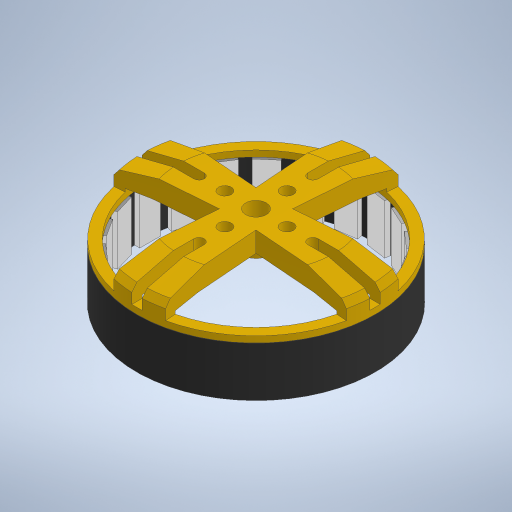
# Autodesk Inventor part: CAN
Saved by Autodesk Inventor 2023.1 (Build 271208000, 208)
## iProperties
Created: 2022-11-08
Part Number: CAN
Material: Generic
Document SubType Name: Modeling
Designer: Nathan Cai
Density: 1 g/cm^3
Appearance: Default
Author: Nathan Cai
Autodesk Inventor part; units mm, degrees
ref_plane "YZ Plane" through (0, 0, 0) normal (1, 0, 0) x (0, 1, 0)
ref_plane "XZ Plane" through (0, 0, 0) normal (0, 1, 0) x (-1, 0, 0)
ref_plane "XY Plane" through (0, 0, 0) normal (0, 0, 1) x (1, 0, 0)
sketch "Sketch1" plane through (0, 0, 0) normal (0, 1, 0) x (-1, 0, 0)
  circle A0 centre (0, 0) radius 23.05
  circle A1 centre (0, 0) radius 21.55
  line L0 (23.05, 0) -> (0, 0) construction
  dimension "d0" = 46.1
  dimension "d1" = 1.5
  constraints: 2 coincident, 2 end point, 1 centre point, 1 horizontal, 1 horizontal alignment, 2 other
extrude "Extrusion1" add sketch "Sketch1" along normal blind 9.6
sketch "Sketch2" plane through (0, 0, 0) normal (0, -1, 0) x (1, 0, 0)
  circle A0 centre (0, 0) radius 21.55 construction
  line L0 (21.55, 0) -> (0, 0) construction
  line L1 (20.457, 2) -> (21.457, 2)
  line L2 (21.457, 2) -> (21.457, -2)
  line L3 (21.457, -2) -> (20.457, -2)
  line L4 (20.457, -2) -> (20.457, 2)
  line L5 (20.457, 2) -> (21.457, -2) construction
  line L6 (21.457, 2) -> (20.457, -2) construction
  line L7 (19.0649, 7.6824) -> (20.0244, 7.9641)
  line L8 (20.0244, 7.9641) -> (21.1513, 4.1261)
  line L9 (21.1513, 4.1261) -> (20.1918, 3.8444)
  line L10 (20.1918, 3.8444) -> (19.0649, 7.6824)
  line L11 (19.0649, 7.6824) -> (21.1513, 4.1261) construction
  line L12 (20.0244, 7.9641) -> (20.1918, 3.8444) construction
  line L13 (16.1282, 12.7424) -> (16.9695, 13.283)
  line L14 (16.9695, 13.283) -> (19.1321, 9.918)
  line L15 (19.1321, 9.918) -> (18.2908, 9.3774)
  line L16 (18.2908, 9.3774) -> (16.1282, 12.7424)
  line L17 (16.1282, 12.7424) -> (19.1321, 9.918) construction
  line L18 (16.9695, 13.283) -> (18.2908, 9.3774) construction
  line L19 (11.885, 16.7701) -> (12.5398, 17.5258)
  line L20 (12.5398, 17.5258) -> (15.5628, 14.9064)
  line L21 (15.5628, 14.9064) -> (14.908, 14.1506)
  line L22 (14.908, 14.1506) -> (11.885, 16.7701)
  line L23 (11.885, 16.7701) -> (15.5628, 14.9064) construction
  line L24 (12.5398, 17.5258) -> (14.908, 14.1506) construction
  line L25 (6.6789, 19.4392) -> (7.0943, 20.3488)
  line L26 (7.0943, 20.3488) -> (10.7328, 18.6871)
  line L27 (10.7328, 18.6871) -> (10.3174, 17.7775)
  line L28 (10.3174, 17.7775) -> (6.6789, 19.4392)
  line L29 (6.6789, 19.4392) -> (10.7328, 18.6871) construction
  line L30 (7.0943, 20.3488) -> (10.3174, 17.7775) construction
  line L31 (0.9317, 20.5334) -> (1.074, 21.5232)
  line L32 (1.074, 21.5232) -> (5.0333, 20.954)
  line L33 (5.0333, 20.954) -> (4.891, 19.9641)
  line L34 (4.891, 19.9641) -> (0.9317, 20.5334)
  line L35 (0.9317, 20.5334) -> (5.0333, 20.954) construction
  line L36 (1.074, 21.5232) -> (4.891, 19.9641) construction
  line L37 (-4.891, 19.9641) -> (-5.0333, 20.954)
  line L38 (-5.0333, 20.954) -> (-1.074, 21.5232)
  line L39 (-1.074, 21.5232) -> (-0.9317, 20.5334)
  line L40 (-0.9317, 20.5334) -> (-4.891, 19.9641)
  line L41 (-4.891, 19.9641) -> (-1.074, 21.5232) construction
  line L42 (-5.0333, 20.954) -> (-0.9317, 20.5334) construction
  line L43 (-10.3174, 17.7775) -> (-10.7328, 18.6871)
  line L44 (-10.7328, 18.6871) -> (-7.0943, 20.3488)
  line L45 (-7.0943, 20.3488) -> (-6.6789, 19.4392)
  line L46 (-6.6789, 19.4392) -> (-10.3174, 17.7775)
  line L47 (-10.3174, 17.7775) -> (-7.0943, 20.3488) construction
  line L48 (-10.7328, 18.6871) -> (-6.6789, 19.4392) construction
  line L49 (-14.908, 14.1506) -> (-15.5628, 14.9064)
  line L50 (-15.5628, 14.9064) -> (-12.5398, 17.5258)
  line L51 (-12.5398, 17.5258) -> (-11.885, 16.7701)
  line L52 (-11.885, 16.7701) -> (-14.908, 14.1506)
  line L53 (-14.908, 14.1506) -> (-12.5398, 17.5258) construction
  line L54 (-15.5628, 14.9064) -> (-11.885, 16.7701) construction
  line L55 (-18.2908, 9.3774) -> (-19.1321, 9.918)
  line L56 (-19.1321, 9.918) -> (-16.9695, 13.283)
  line L57 (-16.9695, 13.283) -> (-16.1282, 12.7424)
  line L58 (-16.1282, 12.7424) -> (-18.2908, 9.3774)
  line L59 (-18.2908, 9.3774) -> (-16.9695, 13.283) construction
  line L60 (-19.1321, 9.918) -> (-16.1282, 12.7424) construction
  line L61 (-20.1918, 3.8444) -> (-21.1513, 4.1261)
  line L62 (-21.1513, 4.1261) -> (-20.0244, 7.9641)
  line L63 (-20.0244, 7.9641) -> (-19.0649, 7.6824)
  line L64 (-19.0649, 7.6824) -> (-20.1918, 3.8444)
  line L65 (-20.1918, 3.8444) -> (-20.0244, 7.9641) construction
  line L66 (-21.1513, 4.1261) -> (-19.0649, 7.6824) construction
  line L67 (-20.457, -2) -> (-21.457, -2)
  line L68 (-21.457, -2) -> (-21.457, 2)
  line L69 (-21.457, 2) -> (-20.457, 2)
  line L70 (-20.457, 2) -> (-20.457, -2)
  line L71 (-20.457, -2) -> (-21.457, 2) construction
  line L72 (-21.457, -2) -> (-20.457, 2) construction
  line L73 (-19.0649, -7.6824) -> (-20.0244, -7.9641)
  line L74 (-20.0244, -7.9641) -> (-21.1513, -4.1261)
  line L75 (-21.1513, -4.1261) -> (-20.1918, -3.8444)
  line L76 (-20.1918, -3.8444) -> (-19.0649, -7.6824)
  line L77 (-19.0649, -7.6824) -> (-21.1513, -4.1261) construction
  line L78 (-20.0244, -7.9641) -> (-20.1918, -3.8444) construction
  line L79 (-16.1282, -12.7424) -> (-16.9695, -13.283)
  line L80 (-16.9695, -13.283) -> (-19.1321, -9.918)
  line L81 (-19.1321, -9.918) -> (-18.2908, -9.3774)
  line L82 (-18.2908, -9.3774) -> (-16.1282, -12.7424)
  line L83 (-16.1282, -12.7424) -> (-19.1321, -9.918) construction
  line L84 (-16.9695, -13.283) -> (-18.2908, -9.3774) construction
  line L85 (-11.885, -16.7701) -> (-12.5398, -17.5258)
  line L86 (-12.5398, -17.5258) -> (-15.5628, -14.9064)
  line L87 (-15.5628, -14.9064) -> (-14.908, -14.1506)
  line L88 (-14.908, -14.1506) -> (-11.885, -16.7701)
  line L89 (-11.885, -16.7701) -> (-15.5628, -14.9064) construction
  line L90 (-12.5398, -17.5258) -> (-14.908, -14.1506) construction
  line L91 (-6.6789, -19.4392) -> (-7.0943, -20.3488)
  line L92 (-7.0943, -20.3488) -> (-10.7328, -18.6871)
  line L93 (-10.7328, -18.6871) -> (-10.3174, -17.7775)
  line L94 (-10.3174, -17.7775) -> (-6.6789, -19.4392)
  line L95 (-6.6789, -19.4392) -> (-10.7328, -18.6871) construction
  line L96 (-7.0943, -20.3488) -> (-10.3174, -17.7775) construction
  line L97 (-0.9317, -20.5334) -> (-1.074, -21.5232)
  line L98 (-1.074, -21.5232) -> (-5.0333, -20.954)
  line L99 (-5.0333, -20.954) -> (-4.891, -19.9641)
  line L100 (-4.891, -19.9641) -> (-0.9317, -20.5334)
  line L101 (-0.9317, -20.5334) -> (-5.0333, -20.954) construction
  line L102 (-1.074, -21.5232) -> (-4.891, -19.9641) construction
  line L103 (4.891, -19.9641) -> (5.0333, -20.954)
  line L104 (5.0333, -20.954) -> (1.074, -21.5232)
  line L105 (1.074, -21.5232) -> (0.9317, -20.5334)
  line L106 (0.9317, -20.5334) -> (4.891, -19.9641)
  line L107 (4.891, -19.9641) -> (1.074, -21.5232) construction
  line L108 (5.0333, -20.954) -> (0.9317, -20.5334) construction
  line L109 (10.3174, -17.7775) -> (10.7328, -18.6871)
  line L110 (10.7328, -18.6871) -> (7.0943, -20.3488)
  line L111 (7.0943, -20.3488) -> (6.6789, -19.4392)
  line L112 (6.6789, -19.4392) -> (10.3174, -17.7775)
  line L113 (10.3174, -17.7775) -> (7.0943, -20.3488) construction
  line L114 (10.7328, -18.6871) -> (6.6789, -19.4392) construction
  line L115 (14.908, -14.1506) -> (15.5628, -14.9064)
  line L116 (15.5628, -14.9064) -> (12.5398, -17.5258)
  line L117 (12.5398, -17.5258) -> (11.885, -16.7701)
  line L118 (11.885, -16.7701) -> (14.908, -14.1506)
  line L119 (14.908, -14.1506) -> (12.5398, -17.5258) construction
  line L120 (15.5628, -14.9064) -> (11.885, -16.7701) construction
  line L121 (18.2908, -9.3774) -> (19.1321, -9.918)
  line L122 (19.1321, -9.918) -> (16.9695, -13.283)
  line L123 (16.9695, -13.283) -> (16.1282, -12.7424)
  line L124 (16.1282, -12.7424) -> (18.2908, -9.3774)
  line L125 (18.2908, -9.3774) -> (16.9695, -13.283) construction
  line L126 (19.1321, -9.918) -> (16.1282, -12.7424) construction
  line L127 (20.1918, -3.8444) -> (21.1513, -4.1261)
  line L128 (21.1513, -4.1261) -> (20.0244, -7.9641)
  line L129 (20.0244, -7.9641) -> (19.0649, -7.6824)
  line L130 (19.0649, -7.6824) -> (20.1918, -3.8444)
  line L131 (20.1918, -3.8444) -> (20.0244, -7.9641) construction
  line L132 (21.1513, -4.1261) -> (19.0649, -7.6824) construction
  point P0 (20.957, 0)
  point P1 (20.6771, 6.0713)
  point P2 (20.1081, 5.9043)
  point P3 (18.129, 11.6508)
  point P4 (17.6301, 11.3302)
  point P5 (14.1122, 16.2864)
  point P6 (13.7239, 15.8382)
  point P7 (8.9522, 19.6026)
  point P8 (8.7058, 19.0632)
  point P9 (3.0669, 21.3307)
  point P10 (2.9825, 20.7437)
  point P11 (-3.0669, 21.3307)
  point P12 (-2.9825, 20.7437)
  point P13 (-8.9522, 19.6026)
  point P14 (-8.7058, 19.0632)
  point P15 (-14.1122, 16.2864)
  point P16 (-13.7239, 15.8382)
  point P17 (-18.129, 11.6508)
  point P18 (-17.6301, 11.3302)
  point P19 (-20.6771, 6.0713)
  point P20 (-20.1081, 5.9043)
  point P21 (-21.55, 0)
  point P22 (-20.957, 0)
  point P23 (-20.6771, -6.0713)
  point P24 (-20.1081, -5.9043)
  point P25 (-18.129, -11.6508)
  point P26 (-17.6301, -11.3302)
  point P27 (-14.1122, -16.2864)
  point P28 (-13.7239, -15.8382)
  point P29 (-8.9522, -19.6026)
  point P30 (-8.7058, -19.0632)
  point P31 (-3.0669, -21.3307)
  point P32 (-2.9825, -20.7437)
  point P33 (3.0669, -21.3307)
  point P34 (2.9825, -20.7437)
  point P35 (8.9522, -19.6026)
  point P36 (8.7058, -19.0632)
  point P37 (14.1122, -16.2864)
  point P38 (13.7239, -15.8382)
  point P39 (18.129, -11.6508)
  point P40 (17.6301, -11.3302)
  point P41 (20.6771, -6.0713)
  point P42 (20.1081, -5.9043)
  dimension "d4" = 1
  dimension "d5" = 4
  dimension "d8" = 360
  constraints: 266 end point, 2 horizontal, 2 midpoint, 2 parallel, 2 point on circle, 1 perpendicular, 1 point on line, 265 other
  measures "d4" distance of L2.end L3.end
  measures "d5" distance of L1.end L2.end
extrude "Extrusion2" add sketch "Sketch2" against normal blind 9.6
sketch "Sketch4" plane through (0, 0, 0) normal (1, 0, 0) x (0, 1, 0)
  line L0 (9.6, 2) -> (9.6, -2) projected
  line L1 (9.6, 0) -> (15.8, 0)
  line L2 (15.8, 0) -> (15.8, 23)
  line L3 (15.8, 23) -> (9.6, 23)
  line L4 (9.6, 23) -> (9.6, 0)
  line L5 (9.6, 0) -> (11.9, 0)
  line L6 (11.9, 0) -> (11.9, 21)
  line L7 (11.9, 21) -> (9.6, 21)
  line L8 (9.6, 21) -> (9.6, 0)
  line L9 (11.4, 21) -> (11.9, 16.3)
  line L10 (9.6, 0) -> (15.8, 0)
  line L11 (15.8, 0) -> (15.8, 3)
  line L12 (15.8, 3) -> (9.6, 3) construction
  line L13 (9.6, 3) -> (9.6, 0)
  line L14 (9.6, 3) -> (11.9, 3.75)
  line L15 (15.8, 0) -> (9.6, 0)
  line L16 (9.6, 0) -> (9.6, 2)
  line L17 (9.6, 2) -> (15.8, 2)
  line L18 (15.8, 2) -> (15.8, 0)
  point P0 (0, 0)
  dimension "d15" = 6.2
  dimension "d16" = 23
  dimension "d17" = 2.3
  dimension "d18" = 21
  dimension "d19" = 1.8
  dimension "d20" = 4.7
  dimension "d28" = 3
  dimension "d29" = 3.75
  dimension "d30" = 2
  constraints: 36 end point, 8 parallel, 4 horizontal, 4 perpendicular, 4 point on line, 1 midpoint
  measures "d15" distance of L3.end L2.end
  measures "d16" distance of L2.end L1.end
  measures "d17" distance of L7.end L6.end
  measures "d18" distance of L6.end L5.end
  measures "d19" distance from line of L4 L9.start
  measures "d20" distance from line of L7 L9.end
  measures "d28" distance of L11.end L10.end
  measures "d29" distance from line of L1 L14.end
  measures "d30" distance of L15.end L0.start
revolve "Revolution1" add sketch "Sketch4" angle 360 about axis through (0, 9.6, 0) along (0, 1, 0) contours L4 L14 L6 L17 | L6 L7 L4 L3 L2 L17 | L7 L6 L9
chamfer "Chamfer1" distance 8 distance2 2 1 edges at (0, 15.8, -23) measured on face at (-1.8348, 15.8, 15.7772)
chamfer "Chamfer2" distance 1 angle 45 1 edges at (0, 13.8, -23)
sketch "Sketch5" plane through (0, 15.8, 0) normal (0, 1, 0) x (1, 0, 0)
  circle A0 centre (0, 0) radius 6 construction
  line L0 (0, 0) -> (0, 6) construction
  circle A1 centre (0, 6) radius 1.25
  circle A2 centre (-6, 0) radius 1.25
  circle A3 centre (0, -6) radius 1.25
  circle A4 centre (6, 0) radius 1.25
  line L1 (-1, 35.1) -> (1, 35.1)
  line L2 (1, 35.1) -> (1, 11)
  line L3 (1, 11) -> (-1, 11) construction
  line L4 (-1, 11) -> (-1, 35.1)
  circle A5 centre (0, 0) radius 23.05 projected
  line L5 (-1, 35.1) -> (1, 11) construction
  line L6 (1, 35.1) -> (-1, 11) construction
  arc A6 (-1, 11) -> (1, 11) centre (0, 11) ccw
  circle A7 centre (0, 0) radius 10 construction
  line L7 (-11, 1) -> (-11, -1) construction
  line L8 (-11, -1) -> (-35.1, -1)
  line L9 (-35.1, -1) -> (-35.1, 1)
  line L10 (-35.1, 1) -> (-11, -1) construction
  line L11 (-35.1, 1) -> (-11, 1)
  line L12 (-35.1, -1) -> (-11, 1) construction
  arc A8 (-11, -1) -> (-11, 1) centre (-11, 0) ccw
  line L13 (-1, -11) -> (1, -11) construction
  line L14 (1, -11) -> (1, -35.1)
  line L15 (1, -35.1) -> (-1, -35.1)
  line L16 (-1, -35.1) -> (1, -11) construction
  line L17 (-1, -35.1) -> (-1, -11)
  line L18 (1, -35.1) -> (-1, -11) construction
  arc A9 (1, -11) -> (-1, -11) centre (0, -11) ccw
  line L19 (11, -1) -> (11, 1) construction
  line L20 (11, 1) -> (35.1, 1)
  line L21 (35.1, 1) -> (35.1, -1)
  line L22 (35.1, -1) -> (11, 1) construction
  line L23 (35.1, -1) -> (11, -1)
  line L24 (35.1, 1) -> (11, -1) construction
  arc A10 (11, 1) -> (11, -1) centre (11, 0) ccw
  line L25 (0, 0) -> (16.2988, 16.2988) construction
  circle A11 centre (0, 0) radius 5 construction
  line L26 (3.5355, 3.5355) -> (22.5012, 5)
  line L27 (3.5355, 3.5355) -> (5, 22.5012)
  arc A12 (3.8726, 7.9001) -> (7.9001, 3.8726) centre (7.6114, 7.6114) ccw
  line L28 (-3.5355, 3.5355) -> (-22.5012, 5)
  line L29 (-3.5355, 3.5355) -> (-5, 22.5012)
  arc A13 (-7.9001, 3.8726) -> (-3.8726, 7.9001) centre (-7.6114, 7.6114) ccw
  line L30 (-3.5355, -3.5355) -> (-5, -22.5012)
  line L31 (-3.5355, -3.5355) -> (-22.5012, -5)
  arc A14 (-3.8726, -7.9001) -> (-7.9001, -3.8726) centre (-7.6114, -7.6114) ccw
  line L32 (3.5355, -3.5355) -> (22.5012, -5)
  line L33 (3.5355, -3.5355) -> (5, -22.5012)
  arc A15 (7.9001, -3.8726) -> (3.8726, -7.9001) centre (7.6114, -7.6114) ccw
  point P0 (0, 23.05)
  point P1 (-23.05, 0)
  point P2 (0, -23.05)
  point P3 (23.05, 0)
  point P4 (-5, -22.5012)
  dimension "d31" = 12
  dimension "d44" = 10
  dimension "d32" = 2.5
  dimension "d35" = 360
  dimension "d37" = 2
  dimension "d38" = 20
  dimension "d41" = 360
  dimension "d43" = 45
  dimension "d45" = 5
  dimension "d46" = 3.75
  dimension "d49" = 360
  constraints: 68 end point, 20 point on circle, 13 centre point, 11 point on line, 4 coincident, 3 midpoint, 2 parallel, 2 tangent, 1 horizontal, 1 perpendicular, 1 vertical, 1 vertical alignment, 105 other
  measures "d32" diameter of A1
  measures "d37" distance of L2.end L3.end
  measures "d38" diameter of A7
  measures "d43" angle of L0 L25
  measures "d45" distance from line of L0 L27.end
  measures "d46" radius of A12
extrude "Extrusion4" cut sketch "Sketch5" against normal blind 5 contours A1 | A2 | A3 | A4 | L1 L2 A5 L4 | A5 L2 A6 L4 | L29 A13 L28 A5 | A5 L26 A12 L27 | L29 L28 A13 | A12 L26 L27 | L11 A8 L8 A5 | A5 L8 L9 L11 | L20 L21 L23 A5 | A5 L23 A10 L20 | L31 A14 L30 A5 | L31 L30 A14 | A5 L33 A15 L32 | L17 A9 L14 A5 | A5 L14 L15 L17 | A15 L33 L32
body "Solid1"
